Autodesk Inventor part; units mm, degrees
(part 2 of 2)
  arc A370 (45.3875, -111.275) -> (45.8875, -111.775) centre (45.8875, -111.275) ccw
  arc A371 (58.8875, -111.775) -> (59.3875, -111.275) centre (58.8875, -111.275) ccw
  line L372 (69.7, -97.775) -> (82.7, -97.775)
  line L373 (69.7, -111.775) -> (82.7, -111.775)
  line L374 (69.2, -98.275) -> (69.2, -111.275)
  line L375 (83.2, -98.275) -> (83.2, -111.275)
  arc A372 (69.7, -97.775) -> (69.2, -98.275) centre (69.7, -98.275) ccw
  arc A373 (83.2, -98.275) -> (82.7, -97.775) centre (82.7, -98.275) ccw
  arc A374 (69.2, -111.275) -> (69.7, -111.775) centre (69.7, -111.275) ccw
  arc A375 (82.7, -111.775) -> (83.2, -111.275) centre (82.7, -111.275) ccw
  line L376 (93.5125, -97.775) -> (106.5125, -97.775)
  line L377 (93.5125, -111.775) -> (106.5125, -111.775)
  line L378 (93.0125, -98.275) -> (93.0125, -111.275)
  line L379 (107.0125, -98.275) -> (107.0125, -111.275)
  arc A376 (93.5125, -97.775) -> (93.0125, -98.275) centre (93.5125, -98.275) ccw
  arc A377 (107.0125, -98.275) -> (106.5125, -97.775) centre (106.5125, -98.275) ccw
  arc A378 (93.0125, -111.275) -> (93.5125, -111.775) centre (93.5125, -111.275) ccw
  arc A379 (106.5125, -111.775) -> (107.0125, -111.275) centre (106.5125, -111.275) ccw
  line L380 (167.3313, -97.775) -> (180.3313, -97.775)
  line L381 (167.3313, -111.775) -> (180.3313, -111.775)
  line L382 (166.8313, -98.275) -> (166.8313, -111.275)
  line L383 (180.8313, -98.275) -> (180.8313, -111.275)
  arc A380 (167.3313, -97.775) -> (166.8313, -98.275) centre (167.3313, -98.275) ccw
  arc A381 (180.8313, -98.275) -> (180.3313, -97.775) centre (180.3313, -98.275) ccw
  arc A382 (166.8313, -111.275) -> (167.3313, -111.775) centre (167.3313, -111.275) ccw
  arc A383 (180.3313, -111.775) -> (180.8313, -111.275) centre (180.3313, -111.275) ccw
  line L384 (220.9563, -98.775) -> (226.7063, -98.775)
  line L385 (220.9563, -112.775) -> (226.7063, -112.775)
  line L386 (220.4563, -99.275) -> (220.4563, -112.275)
  line L387 (227.2063, -99.275) -> (227.2063, -112.275)
  arc A384 (220.9563, -98.775) -> (220.4563, -99.275) centre (220.9563, -99.275) ccw
  arc A385 (227.2063, -99.275) -> (226.7063, -98.775) centre (226.7063, -99.275) ccw
  arc A386 (220.4563, -112.275) -> (220.9563, -112.775) centre (220.9563, -112.275) ccw
  arc A387 (226.7063, -112.775) -> (227.2063, -112.275) centre (226.7063, -112.275) ccw
  line L388 (120.9562, -98.775) -> (126.7063, -98.775)
  line L389 (120.9562, -112.775) -> (126.7063, -112.775)
  line L390 (120.4563, -99.275) -> (120.4563, -112.275)
  line L391 (127.2062, -99.275) -> (127.2062, -112.275)
  arc A388 (120.9562, -98.775) -> (120.4563, -99.275) centre (120.9562, -99.275) ccw
  arc A389 (127.2062, -99.275) -> (126.7063, -98.775) centre (126.7063, -99.275) ccw
  arc A390 (120.4563, -112.275) -> (120.9562, -112.775) centre (120.9562, -112.275) ccw
  arc A391 (126.7063, -112.775) -> (127.2062, -112.275) centre (126.7063, -112.275) ccw
  line L392 (238.7688, -97.775) -> (251.7687, -97.775)
  line L393 (238.7688, -111.775) -> (251.7687, -111.775)
  line L394 (238.2688, -98.275) -> (238.2688, -111.275)
  line L395 (252.2688, -98.275) -> (252.2688, -111.275)
  arc A392 (238.7688, -97.775) -> (238.2688, -98.275) centre (238.7688, -98.275) ccw
  arc A393 (252.2688, -98.275) -> (251.7687, -97.775) centre (251.7687, -98.275) ccw
  arc A394 (238.2688, -111.275) -> (238.7688, -111.775) centre (238.7688, -111.275) ccw
  arc A395 (251.7687, -111.775) -> (252.2688, -111.275) centre (251.7687, -111.275) ccw
  line L396 (264.9625, -97.775) -> (277.9625, -97.775)
  line L397 (264.9625, -111.775) -> (277.9625, -111.775)
  line L398 (264.4625, -98.275) -> (264.4625, -111.275)
  line L399 (278.4625, -98.275) -> (278.4625, -111.275)
  arc A396 (264.9625, -97.775) -> (264.4625, -98.275) centre (264.9625, -98.275) ccw
  arc A397 (278.4625, -98.275) -> (277.9625, -97.775) centre (277.9625, -98.275) ccw
  arc A398 (264.4625, -111.275) -> (264.9625, -111.775) centre (264.9625, -111.275) ccw
  arc A399 (277.9625, -111.775) -> (278.4625, -111.275) centre (277.9625, -111.275) ccw
  line L400 (288.775, -97.775) -> (301.775, -97.775)
  line L401 (288.775, -111.775) -> (301.775, -111.775)
  line L402 (288.275, -98.275) -> (288.275, -111.275)
  line L403 (302.275, -98.275) -> (302.275, -111.275)
  arc A400 (288.775, -97.775) -> (288.275, -98.275) centre (288.775, -98.275) ccw
  arc A401 (302.275, -98.275) -> (301.775, -97.775) centre (301.775, -98.275) ccw
  arc A402 (288.275, -111.275) -> (288.775, -111.775) centre (288.775, -111.275) ccw
  arc A403 (301.775, -111.775) -> (302.275, -111.275) centre (301.775, -111.275) ccw
  line L404 (307.825, -97.775) -> (320.825, -97.775)
  line L405 (307.825, -111.775) -> (320.825, -111.775)
  line L406 (307.325, -98.275) -> (307.325, -111.275)
  line L407 (321.325, -98.275) -> (321.325, -111.275)
  arc A404 (307.825, -97.775) -> (307.325, -98.275) centre (307.825, -98.275) ccw
  arc A405 (321.325, -98.275) -> (320.825, -97.775) centre (320.825, -98.275) ccw
  arc A406 (307.325, -111.275) -> (307.825, -111.775) centre (307.825, -111.275) ccw
  arc A407 (320.825, -111.775) -> (321.325, -111.275) centre (320.825, -111.275) ccw
  line L408 (326.875, -97.775) -> (339.875, -97.775)
  line L409 (326.875, -111.775) -> (339.875, -111.775)
  line L410 (326.375, -98.275) -> (326.375, -111.275)
  line L411 (340.375, -98.275) -> (340.375, -111.275)
  arc A408 (326.875, -97.775) -> (326.375, -98.275) centre (326.875, -98.275) ccw
  arc A409 (340.375, -98.275) -> (339.875, -97.775) centre (339.875, -98.275) ccw
  arc A410 (326.375, -111.275) -> (326.875, -111.775) centre (326.875, -111.275) ccw
  arc A411 (339.875, -111.775) -> (340.375, -111.275) centre (339.875, -111.275) ccw
  line L412 (0, 0) -> (342.9, 0)
  line L413 (0, -114.3) -> (342.9, -114.3)
  line L414 (0, 0) -> (0, -114.3)
  line L415 (342.9, 0) -> (342.9, -114.3)
  point P0 (207.3125, -73.175)
  point P1 (207.3125, -60.175)
  point P2 (226.3625, -73.175)
  point P3 (226.3625, -60.175)
  point P4 (278.4625, -60.175)
  point P5 (278.4625, -73.175)
  point P6 (16.525, -79.225)
  point P7 (16.525, -92.225)
  point P8 (16.025, -92.725)
  point P9 (3.025, -92.725)
  point P10 (35.075, -92.725)
  point P11 (22.075, -92.725)
  point P12 (66.0312, -92.725)
  point P13 (53.0313, -92.725)
  point P14 (96.9875, -92.725)
  point P15 (83.9875, -92.725)
  point P16 (83.4875, -92.225)
  point P17 (83.4875, -79.225)
  point P18 (116.0375, -92.725)
  point P19 (103.0375, -92.725)
  point P20 (135.0875, -92.725)
  point P21 (122.0875, -92.725)
  point P22 (154.6375, -79.225)
  point P23 (154.6375, -92.225)
  point P24 (154.1375, -92.725)
  point P25 (141.1375, -92.725)
  point P26 (173.1875, -92.725)
  point P27 (160.1875, -92.725)
  point P28 (192.2375, -92.725)
  point P29 (179.2375, -92.725)
  point P30 (211.2875, -92.725)
  point P31 (198.2875, -92.725)
  point P32 (197.7875, -92.225)
  point P33 (197.7875, -79.225)
  point P34 (230.3375, -92.725)
  point P35 (217.3375, -92.725)
  point P36 (216.8375, -92.225)
  point P37 (216.8375, -79.225)
  point P38 (249.3875, -92.725)
  point P39 (236.3875, -92.725)
  point P40 (268.4375, -92.725)
  point P41 (255.4375, -92.725)
  point P42 (295.1313, -79.225)
  point P43 (295.1313, -92.225)
  point P44 (294.6313, -92.725)
  point P45 (281.6313, -92.725)
  point P46 (320.825, -92.725)
  point P47 (307.825, -92.725)
  point P48 (307.325, -92.225)
  point P49 (307.325, -79.225)
  point P50 (339.875, -92.725)
  point P51 (326.875, -92.725)
  point P52 (3.025, -97.775)
  point P53 (16.025, -97.775)
  point P54 (16.525, -98.275)
  point P55 (16.525, -111.275)
  point P56 (22.075, -97.775)
  point P57 (35.075, -97.775)
  point P58 (45.8875, -97.775)
  point P59 (58.8875, -97.775)
  point P60 (69.7, -97.775)
  point P61 (82.7, -97.775)
  point P62 (83.2, -98.275)
  point P63 (83.2, -111.275)
  point P64 (93.5125, -97.775)
  point P65 (106.5125, -97.775)
  point P66 (93.0125, -111.275)
  point P67 (93.0125, -98.275)
  point P68 (167.3313, -97.775)
  point P69 (180.3313, -97.775)
  point P70 (127.2063, -99.275)
  point P71 (127.2063, -112.275)
  point P72 (120.4562, -112.275)
  point P73 (120.4562, -99.275)
  point P74 (238.7688, -97.775)
  point P75 (251.7687, -97.775)
  point P76 (264.9625, -97.775)
  point P77 (277.9625, -97.775)
  point P78 (278.4625, -98.275)
  point P79 (278.4625, -111.275)
  point P80 (288.775, -97.775)
  point P81 (301.775, -97.775)
  point P82 (307.825, -97.775)
  point P83 (320.825, -97.775)
  point P84 (307.325, -111.275)
  point P85 (307.325, -98.275)
  point P86 (326.875, -97.775)
  point P87 (339.875, -97.775)
  point P88 (263.675, -16.525)
  point P89 (250.675, -16.525)
  point P90 (282.725, -16.525)
  point P91 (269.725, -16.525)
  point P92 (301.775, -16.525)
  point P93 (288.775, -16.525)
  point P94 (320.825, -16.525)
  point P95 (307.825, -16.525)
  point P96 (307.325, -16.025)
  point P97 (307.325, -3.025)
  point P98 (339.875, -16.525)
  point P99 (326.875, -16.525)
  point P100 (16.525, -22.075)
  point P101 (16.525, -35.075)
  point P102 (92.725, -22.075)
  point P103 (92.725, -35.075)
  point P104 (97.775, -35.075)
  point P105 (97.775, -22.075)
  point P106 (207.025, -22.075)
  point P107 (207.025, -35.075)
  point P108 (313.863, -22.575)
  point P109 (319.613, -22.575)
  point P110 (289.987, -22.575)
  point P111 (295.737, -22.575)
  point P112 (16.525, -41.125)
  point P113 (16.525, -54.125)
  point P114 (83.2, -41.125)
  point P115 (83.2, -54.125)
  point P116 (88.25, -54.125)
  point P117 (88.25, -41.125)
  point P118 (197.5, -41.125)
  point P119 (197.5, -54.125)
  point P120 (216.55, -41.125)
  point P121 (216.55, -54.125)
  point P122 (316.5625, -41.125)
  point P123 (316.5625, -54.125)
  point P124 (16.525, -60.175)
  point P125 (16.525, -73.175)
  point P126 (47.7688, -73.175)
  point P127 (47.7688, -60.175)
  point P128 (87.9625, -60.175)
  point P129 (87.9625, -73.175)
  point P130 (93.0125, -73.175)
  point P131 (93.0125, -60.175)
  point P132 (92.725, -3.025)
  point P133 (92.725, -16.025)
  point P134 (92.225, -16.525)
  point P135 (79.225, -16.525)
  point P136 (16.525, -3.025)
  point P137 (16.525, -16.025)
  point P138 (16.025, -16.525)
  point P139 (3.025, -16.525)
  point P140 (155.425, -16.525)
  point P141 (97.775, -3.025)
  point P142 (187.475, -16.525)
  point P143 (174.475, -16.525)
  point P144 (207.025, -3.025)
  point P145 (207.025, -16.025)
  point P146 (225.575, -16.525)
  point P147 (54.125, -16.525)
  point P148 (41.125, -16.525)
  point P149 (130.325, -16.525)
  point P150 (117.325, -16.525)
  constraints: 832 end point, 824 point on circle, 412 centre point
extrude "Extrusion1" add sketch "Sketch1" along normal blind 5
sketch "Sketch2" plane through (342.9, -114.3, 0) normal (1, 0, 0) x (0, 0, -1)
  line L0 (0, 114.3) -> (-5, 114.3) projected
  line L1 (-5, 114.3) -> (-5, 0) projected
  line L2 (0, 114.3) -> (-5, 114.3)
  line L3 (-5, 114.3) -> (-5, 0)
  line L4 (-5, 0) -> (0, 0)
  line L5 (0, 0) -> (0, 114.3)
  constraints: 8 end point, 2 parallel, 1 horizontal, 1 perpendicular
extrude "Extrusion2" add sketch "Sketch2" along normal blind 23.432
sketch "Sketch3" plane through (0, 0, 0) normal (0, 1, 0) x (1, 0, 0)
  line L0 (366.332, -5) -> (366.332, 0) projected
  line L1 (0, -5) -> (366.332, -5) projected
  line L2 (366.332, 0) -> (332.994, 0)
  line L3 (332.994, -5) -> (366.332, -5)
  line L4 (366.332, -5) -> (366.332, 0)
  line L5 (0, 0) -> (0, -5) projected
  line L6 (332.994, 0) -> (0, 0)
  line L7 (0, 0) -> (0, -5)
  line L8 (0, -5) -> (332.994, -5)
  dimension "d4" = 33.338
  constraints: 12 end point, 2 horizontal, 2 parallel, 1 perpendicular, 1 point on line
  measures "d4" distance of L3.end L3.start
extrude "Extrusion3" add sketch "Sketch3" along normal blind 9.525
sketch "Sketch4" plane through (0, -114.3, 0) normal (-1, 0, 0) x (0, 0, 1)
  line L0 (0, 123.825) -> (5, 123.825) projected
  line L1 (5, 114.3) -> (5, 0) projected
  line L2 (0, 123.825) -> (5, 123.825)
  line L3 (5, 123.825) -> (5, 0)
  line L4 (5, 0) -> (0, 0)
  line L5 (0, 0) -> (0, 123.825)
  point P0 (0, 114.3)
  constraints: 8 end point, 2 parallel, 1 horizontal, 1 perpendicular
extrude "Extrusion4" add sketch "Sketch4" along normal blind 9.906
equation "\"BendRadius\" = Thickness"
equation "\"BendReliefWidth\" = Thickness"
equation "\"BendReliefDepth\" = 0.5 * Thickness"
equation "\"CornerReliefSize\" = 4 * Thickness"
equation "\"MinimumRemnant\" = 2 * Thickness"
equation "\"TransitionRadius\" = BendRadius"
equation "\"JacobiRadiusSize\" = BendRadius"
equation "\"GapSize\" = Thickness"
equation "\"Thickness\" = 0.5"
body "Solid1"
